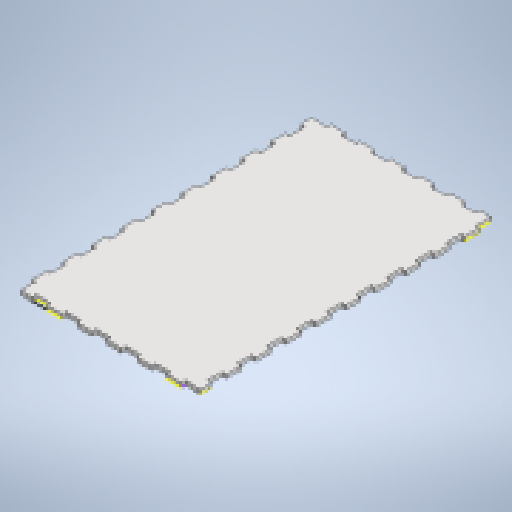
# Autodesk Inventor part: ground
Saved by Autodesk Inventor 2025.3 (Build 293356000, 356)
## iProperties
Created: 2025-12-07
Part Number: ground
Material: Generic
Document SubType Name: Modeling
Designer: hazem
Density: 1 g/cm^3
Appearance: Default
Author: hazem
Autodesk Inventor part; units mm, degrees
ref_plane "YZ Plane" through (0, 0, 0) normal (1, 0, 0) x (0, 1, 0)
ref_plane "XZ Plane" through (0, 0, 0) normal (0, 1, 0) x (-1, 0, 0)
ref_plane "XY Plane" through (0, 0, 0) normal (0, 0, 1) x (1, 0, 0)
sketch "Sketch1" plane through (0, 0, 0) normal (0, 1, 0) x (-1, 0, 0)
  line L0 (58.4588, 59.1887) -> (-121.5412, 59.1887)
  line L1 (-121.5412, -240.8113) -> (58.4588, -240.8113)
  line L2 (58.4588, -240.8113) -> (58.4588, 59.1887)
  line L3 (-121.5412, 59.1887) -> (-121.5412, -240.8113)
  line L4 (58.4588, 59.1887) -> (54.4588, 59.1887)
  line L5 (54.4588, 59.1887) -> (54.4588, 44.1887)
  line L6 (54.4588, 44.1887) -> (58.4588, 44.1887)
  line L7 (58.4588, 44.1887) -> (58.4588, 59.1887)
  line L8 (54.4588, 29.1887) -> (54.4588, 14.1887)
  line L9 (54.4588, 14.1887) -> (58.4588, 14.1887)
  line L10 (58.4588, 29.1887) -> (54.4588, 29.1887)
  line L11 (54.4588, -0.8113) -> (54.4588, -15.8113)
  line L12 (54.4588, -15.8113) -> (58.4588, -15.8113)
  line L13 (58.4588, -0.8113) -> (54.4588, -0.8113)
  line L14 (54.4588, -30.8113) -> (54.4588, -45.8113)
  line L15 (54.4588, -45.8113) -> (58.4588, -45.8113)
  line L16 (58.4588, -30.8113) -> (54.4588, -30.8113)
  line L17 (54.4588, -60.8113) -> (54.4588, -75.8113)
  line L18 (54.4588, -75.8113) -> (58.4588, -75.8113)
  line L19 (58.4588, -60.8113) -> (54.4588, -60.8113)
  line L20 (54.4588, -90.8113) -> (54.4588, -105.8113)
  line L21 (54.4588, -105.8113) -> (58.4588, -105.8113)
  line L22 (58.4588, -90.8113) -> (54.4588, -90.8113)
  line L23 (54.4588, -120.8113) -> (54.4588, -135.8113)
  line L24 (54.4588, -135.8113) -> (58.4588, -135.8113)
  line L25 (58.4588, -120.8113) -> (54.4588, -120.8113)
  line L26 (54.4588, -150.8113) -> (54.4588, -165.8113)
  line L27 (54.4588, -165.8113) -> (58.4588, -165.8113)
  line L28 (58.4588, -150.8113) -> (54.4588, -150.8113)
  line L29 (54.4588, -180.8113) -> (54.4588, -195.8113)
  line L30 (54.4588, -195.8113) -> (58.4588, -195.8113)
  line L31 (58.4588, -180.8113) -> (54.4588, -180.8113)
  line L32 (54.4588, -210.8113) -> (54.4588, -225.8113)
  line L33 (54.4588, -225.8113) -> (58.4588, -225.8113)
  line L34 (58.4588, -210.8113) -> (54.4588, -210.8113)
  line L35 (-121.5412, -240.8113) -> (-117.5412, -240.8113)
  line L36 (-117.5412, -240.8113) -> (-117.5412, -225.8113)
  line L37 (-117.5412, -225.8113) -> (-121.5412, -225.8113)
  line L38 (-121.5412, -225.8113) -> (-121.5412, -240.8113)
  line L39 (-117.5412, -210.8113) -> (-117.5412, -195.8113)
  line L40 (-117.5412, -195.8113) -> (-121.5412, -195.8113)
  line L41 (-121.5412, -210.8113) -> (-117.5412, -210.8113)
  line L42 (-117.5412, -180.8113) -> (-117.5412, -165.8113)
  line L43 (-117.5412, -165.8113) -> (-121.5412, -165.8113)
  line L44 (-121.5412, -180.8113) -> (-117.5412, -180.8113)
  line L45 (-117.5412, -150.8113) -> (-117.5412, -135.8113)
  line L46 (-117.5412, -135.8113) -> (-121.5412, -135.8113)
  line L47 (-121.5412, -150.8113) -> (-117.5412, -150.8113)
  line L48 (-117.5412, -120.8113) -> (-117.5412, -105.8113)
  line L49 (-117.5412, -105.8113) -> (-121.5412, -105.8113)
  line L50 (-121.5412, -120.8113) -> (-117.5412, -120.8113)
  line L51 (-117.5412, -90.8113) -> (-117.5412, -75.8113)
  line L52 (-117.5412, -75.8113) -> (-121.5412, -75.8113)
  line L53 (-121.5412, -90.8113) -> (-117.5412, -90.8113)
  line L54 (-117.5412, -60.8113) -> (-117.5412, -45.8113)
  line L55 (-117.5412, -45.8113) -> (-121.5412, -45.8113)
  line L56 (-121.5412, -60.8113) -> (-117.5412, -60.8113)
  line L57 (-117.5412, -30.8113) -> (-117.5412, -15.8113)
  line L58 (-117.5412, -15.8113) -> (-121.5412, -15.8113)
  line L59 (-121.5412, -30.8113) -> (-117.5412, -30.8113)
  line L60 (-117.5412, -0.8113) -> (-117.5412, 14.1887)
  line L61 (-117.5412, 14.1887) -> (-121.5412, 14.1887)
  line L62 (-121.5412, -0.8113) -> (-117.5412, -0.8113)
  line L63 (-117.5412, 29.1887) -> (-117.5412, 44.1887)
  line L64 (-117.5412, 44.1887) -> (-121.5412, 44.1887)
  line L65 (-121.5412, 29.1887) -> (-117.5412, 29.1887)
  line L66 (58.4588, -240.8113) -> (43.4588, -240.8113)
  line L67 (43.4588, -240.8113) -> (43.4588, -236.8113)
  line L68 (43.4588, -236.8113) -> (58.4588, -236.8113)
  line L69 (58.4588, -236.8113) -> (58.4588, -240.8113)
  line L70 (13.4588, -236.8113) -> (28.4588, -236.8113)
  line L71 (13.4588, -240.8113) -> (13.4588, -236.8113)
  line L72 (28.4588, -236.8113) -> (28.4588, -240.8113)
  line L73 (-16.5412, -236.8113) -> (-1.5412, -236.8113)
  line L74 (-16.5412, -240.8113) -> (-16.5412, -236.8113)
  line L75 (-1.5412, -236.8113) -> (-1.5412, -240.8113)
  line L76 (-46.5412, -236.8113) -> (-31.5412, -236.8113)
  line L77 (-46.5412, -240.8113) -> (-46.5412, -236.8113)
  line L78 (-31.5412, -236.8113) -> (-31.5412, -240.8113)
  line L79 (-76.5412, -236.8113) -> (-61.5412, -236.8113)
  line L80 (-76.5412, -240.8113) -> (-76.5412, -236.8113)
  line L81 (-61.5412, -236.8113) -> (-61.5412, -240.8113)
  line L82 (-106.5412, -236.8113) -> (-91.5412, -236.8113)
  line L83 (-106.5412, -240.8113) -> (-106.5412, -236.8113)
  line L84 (-91.5412, -236.8113) -> (-91.5412, -240.8113)
  line L85 (-121.5412, 59.1887) -> (-106.5412, 59.1887)
  line L86 (-106.5412, 59.1887) -> (-106.5412, 55.1887)
  line L87 (-106.5412, 55.1887) -> (-121.5412, 55.1887)
  line L88 (-121.5412, 55.1887) -> (-121.5412, 59.1887)
  line L89 (-76.5412, 59.1887) -> (-76.5412, 55.1887)
  line L90 (-76.5412, 55.1887) -> (-91.5412, 55.1887)
  line L91 (-91.5412, 55.1887) -> (-91.5412, 59.1887)
  line L92 (-46.5412, 59.1887) -> (-46.5412, 55.1887)
  line L93 (-46.5412, 55.1887) -> (-61.5412, 55.1887)
  line L94 (-61.5412, 55.1887) -> (-61.5412, 59.1887)
  line L95 (-16.5412, 59.1887) -> (-16.5412, 55.1887)
  line L96 (-16.5412, 55.1887) -> (-31.5412, 55.1887)
  line L97 (-31.5412, 55.1887) -> (-31.5412, 59.1887)
  line L98 (13.4588, 59.1887) -> (13.4588, 55.1887)
  line L99 (13.4588, 55.1887) -> (-1.5412, 55.1887)
  line L100 (-1.5412, 55.1887) -> (-1.5412, 59.1887)
  line L101 (43.4588, 59.1887) -> (43.4588, 55.1887)
  line L102 (43.4588, 55.1887) -> (28.4588, 55.1887)
  line L103 (28.4588, 55.1887) -> (28.4588, 59.1887)
  dimension "d22" = 4
  dimension "d23" = 15
  dimension "d26" = 30
  dimension "d31" = 4
  dimension "d32" = 15
  dimension "d35" = 30
  dimension "d40" = 15
  dimension "d41" = 4
  dimension "d44" = 30
  dimension "d49" = 15
  dimension "d50" = 4
  dimension "d53" = 30
  constraints: 204 end point, 36 vertical alignment, 27 parallel, 9 collinear, 8 horizontal, 4 perpendicular, 1 vertical, 139 other
  measures "d22" distance of L6.end L5.end
  measures "d23" distance of L5.end L4.end
  measures "d26" distance of L4.end L8.start
  measures "d31" distance of L37.end L36.end
  measures "d32" distance of L36.end L35.end
  measures "d35" distance of L35.end L39.start
  measures "d40" distance of L67.end L68.end
  measures "d41" distance of L66.end L67.end
  measures "d44" distance of L67.end L70.start
  measures "d49" distance of L86.end L87.end
  measures "d50" distance of L85.end L86.end
  measures "d53" distance of L85.end L89.start
extrude "Extrusion1" add sketch "Sketch1" along normal blind 4 contours L5 L6 L2 L10 L8 L9 L13 L11 L12 L16 L14 L15 L19 L17 L18 L22 L20 L21 L25 L23 L24 L28 L26 L27 L31 L29 L30 L34 L32 L33 L68 L67 L1 L72 L70 L71 L75 L73 L74 L78 L76 L77 L81 L79 L80 L84 L82 L83 L36 L37 L3 L41 L39 L40 L44 L42 L43 L47 L45 L46 L50 L48 L49 L53 L51 L52 L56 L54 L55 L59 L57 L58 L62 L60 L61 L65 L63 L64 L87 L86 L0 L91 L90 L89 L94 L93 L92 L97 L96 L95 L100 L99 L98 L103 L102 L101
sketch "Sketch2" plane through (0, 0, 0) normal (0, -1, 0) x (1, 0, 0)
  line L0 (-54.4588, 29.1887) -> (-58.4588, 29.1887) projected
  line L1 (-58.4588, 29.1887) -> (-58.4588, 44.1887) projected
  line L2 (-54.4588, 29.1887) -> (-58.4588, 29.1887)
  line L3 (-58.4588, 29.1887) -> (-58.4588, 44.1887)
  line L4 (-58.4588, 44.1887) -> (-54.4588, 44.1887)
  line L5 (-54.4588, 44.1887) -> (-54.4588, 29.1887)
  line L6 (91.5412, 59.1887) -> (106.5412, 59.1887) projected
  line L7 (91.5412, 59.1887) -> (106.5412, 59.1887)
  line L8 (106.5412, 59.1887) -> (106.5412, 55.1887)
  line L9 (106.5412, 55.1887) -> (91.5412, 55.1887)
  line L10 (91.5412, 55.1887) -> (91.5412, 59.1887)
  line L11 (117.5412, -225.8113) -> (117.5412, -240.8113) projected
  line L12 (106.5412, -236.8113) -> (91.5412, -236.8113) projected
  line L13 (117.5412, -240.8113) -> (106.5412, -240.8113)
  line L14 (106.5412, -240.8113) -> (106.5412, -236.8113)
  line L15 (106.5412, -236.8113) -> (117.5412, -236.8113)
  line L16 (117.5412, -236.8113) -> (117.5412, -240.8113)
  line L17 (121.5412, -225.8113) -> (117.5412, -225.8113) projected
  line L18 (121.5412, -210.8113) -> (121.5412, -225.8113) projected
  line L19 (117.5412, -225.8113) -> (121.5412, -225.8113)
  line L20 (121.5412, -225.8113) -> (121.5412, -210.8113)
  line L21 (121.5412, -210.8113) -> (117.5412, -210.8113)
  line L22 (117.5412, -210.8113) -> (117.5412, -225.8113)
  line L23 (-54.4588, -225.8113) -> (-54.4588, -210.8113) projected
  line L24 (-54.4588, -225.8113) -> (-58.4588, -225.8113)
  line L25 (-58.4588, -225.8113) -> (-58.4588, -236.8113)
  line L26 (-58.4588, -236.8113) -> (-54.4588, -236.8113)
  line L27 (-54.4588, -236.8113) -> (-54.4588, -225.8113)
  line L28 (-28.4588, -240.8113) -> (-43.4588, -240.8113) projected
  line L29 (-43.4588, -240.8113) -> (-43.4588, -236.8113) projected
  line L30 (-28.4588, -240.8113) -> (-43.4588, -240.8113)
  line L31 (-43.4588, -240.8113) -> (-43.4588, -236.8113)
  line L32 (-43.4588, -236.8113) -> (-28.4588, -236.8113)
  line L33 (-28.4588, -236.8113) -> (-28.4588, -240.8113)
  line L34 (121.5412, 55.1887) -> (121.5412, 44.1887) projected
  line L35 (121.5412, 44.1887) -> (117.5412, 44.1887) projected
  line L36 (121.5412, 55.1887) -> (117.5412, 55.1887)
  line L37 (117.5412, 55.1887) -> (117.5412, 44.1887)
  line L38 (117.5412, 44.1887) -> (121.5412, 44.1887)
  line L39 (121.5412, 44.1887) -> (121.5412, 55.1887)
  line L40 (-54.4588, 59.1887) -> (-43.4588, 59.1887) projected
  line L41 (-43.4588, 55.1887) -> (-28.4588, 55.1887) projected
  line L42 (-54.4588, 59.1887) -> (-43.4588, 59.1887)
  line L43 (-43.4588, 59.1887) -> (-43.4588, 55.1887)
  line L44 (-43.4588, 55.1887) -> (-54.4588, 55.1887)
  line L45 (-54.4588, 55.1887) -> (-54.4588, 59.1887)
  point P0 (0, 0)
  constraints: 64 end point, 16 parallel, 8 horizontal, 8 perpendicular
extrude "Extrusion2" cut sketch "Sketch2" against normal through all
equation "\"d22\" = WoodThickness"
equation "\"d26\" = 2 * d23"
equation "\"d31\" = WoodThickness"
equation "\"d35\" = 2 * d32"
equation "\"d41\" = WoodThickness"
equation "\"d44\" = 2 * d40"
equation "\"d50\" = WoodThickness"
equation "\"d53\" = 2 * d49"
equation "\"d2\" = WoodThickness"
equation "\"WoodThickness\" = 4"
body "Solid1"
